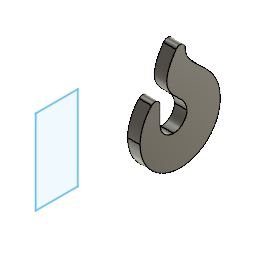
firesim-logo v1 (Autodesk Fusion 360 design; units mm, degrees)
Autodesk Fusion 360 part; units mm, degrees
sketch "Sketch4" plane through (0, 0, 0) normal (1, 0, 0) x (0, 1, 0)
  line L0 (-43.5755, -0.0599) -> (-23.5755, -0.0599)
  line L1 (-23.5755, -0.0599) -> (-23.5755, -40.0599)
  line L2 (-23.5755, -40.0599) -> (-43.5755, -40.0599)
  line L3 (-43.5755, -40.0599) -> (-43.5755, -0.0599)
  dimension "d3" = 20
  dimension "d4" = 40
  constraint horizontal L0
  constraint vertical L1
  constraint horizontal L2
  constraint vertical L3
  measures "d3" distance of L0.start L0.end
  measures "d4" distance of L0.start L2.end
sketch "Sketch6" plane through (0, 0, 0) normal (1, 0, 0) x (0, 1, 0)
  spline S0 degree 3 poles (21.4313, -2.3672) (21.4313, -0.0056) (18.3899, 0.8837) (17.0508, -1.0735) knots 0 0 0 0 1 1 1 1
  spline S1 degree 3 poles (17.0508, -1.0735) (4.7625, -19.0352) (22.225, -19.8438) (22.225, -28.575) knots 0 0 0 0 1 1 1 1
  spline S2 degree 3 poles (22.225, -28.575) (22.225, -32.1101) (19.3363, -34.9704) (15.7907, -34.9244) knots 0 0 0 0 1 1 1 1
  spline S3 degree 3 poles (15.7907, -34.9244) (12.3011, -34.8792) (9.525, -31.9703) (9.525, -28.4803) knots 0 0 0 0 1 1 1 1
  line L0 (9.525, -28.4803) -> (9.525, -19.9961)
  spline S4 degree 3 poles (9.525, -19.9961) (9.525, -17.8428) (6.8986, -16.7988) (5.4142, -18.3586) knots 0 0 0 0 1 1 1 1
  spline S5 degree 3 poles (5.4142, -18.3586) (2.7584, -21.1493) (0, -25.929) (0, -31.75) knots 0 0 0 0 1 1 1 1
  spline S6 degree 3 poles (0, -31.75) (0, -42.2542) (8.5458, -50.8) (19.05, -50.8) knots 0 0 0 0 1 1 1 1
  spline S7 degree 3 poles (19.05, -50.8) (29.5542, -50.8) (38.1, -42.2542) (38.1, -31.75) knots 0 0 0 0 1 1 1 1
  spline S8 degree 3 poles (38.1, -31.75) (38.1, -14.854) (21.4313, -12.6005) (21.4313, -2.3672) knots 0 0 0 0 1 1 1 1
extrude "Extrude1" add sketch "Sketch6" along normal blind 6
